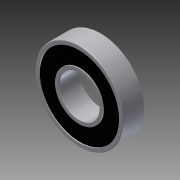
# Autodesk Inventor part: R10-2RS
Saved by Autodesk Inventor 2013 (Build 170138000, 138)
## iProperties
Created: 2013-04-02
Part Number: R10-2RS
Material: Generic
Document SubType Name: Modeling
Designer: mvarma
Density: 1 g/cm^3
Author: mvarma
Autodesk Inventor part; units mm, degrees
ref_plane "YZ Plane" through (0, 0, 0) normal (1, 0, 0) x (0, 1, 0)
ref_plane "XZ Plane" through (0, 0, 0) normal (0, 1, 0) x (-1, 0, 0)
ref_plane "XY Plane" through (0, 0, 0) normal (0, 0, 1) x (1, 0, 0)
sketch "Sketch1" plane through (0, 0, 0) normal (0, 0, 1) x (1, 0, 0)
  circle A0 centre (0, 0) radius 17.4625
  circle A1 centre (0, 0) radius 15.875
  circle A2 centre (0, 0) radius 7.9375
  circle A3 centre (0, 0) radius 9.525
  dimension "d0" = 34.925
  dimension "d2" = 31.75
  dimension "d3" = 15.875
  dimension "d4" = 19.05
  constraints: 4 centre point, 4 coincident
  measures "d0" diameter of A0
  measures "d2" diameter of A1
  measures "d3" diameter of A2
  measures "d4" diameter of A3
extrude "Extrusion1" add sketch "Sketch1" along normal blind 4.3656 contours A0 | A1 | A3
extrude "Extrusion2" cut sketch "Sketch1" along normal blind 0.3969 contours A1
fillet "Fillet1" radius 0.3969 2 edges at (-17.4625, 0, 0) (-7.9375, 0, 0)
mirror "Mirror1" about plane through (0, 0, 4.3656) normal (0, 0, 1)
body "Solid1"
